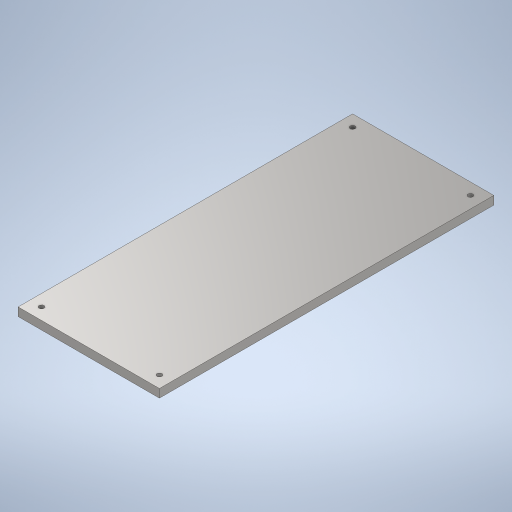
# Autodesk Inventor part: Tutup_system
Saved by Autodesk Inventor 2023.1 (Build 271208000, 208)
## iProperties
Created: 2024-03-27
Part Number: Tutup_system
Material: Generic
Document SubType Name: Modeling
Designer: bahariridwan
Density: 1 g/cm^3
Appearance: Stainless - Brushed
Author: bahariridwan
Autodesk Inventor part; units mm, degrees
ref_plane "YZ Plane" through (0, 0, 0) normal (1, 0, 0) x (0, 1, 0)
ref_plane "XZ Plane" through (0, 0, 0) normal (0, 1, 0) x (-1, 0, 0)
ref_plane "XY Plane" through (0, 0, 0) normal (0, 0, 1) x (1, 0, 0)
sketch "Sketch1" plane through (0, 0, 0) normal (0, 1, 0) x (-1, 0, 0)
  line L0 (0, 0) -> (84.487, 0)
  line L1 (84.487, 0) -> (84.487, -200)
  line L2 (84.487, -200) -> (0, -200)
  line L3 (0, -200) -> (0, 0)
  constraints: 8 end point, 2 parallel, 1 horizontal, 1 perpendicular
extrude "Extrusion1" add sketch "Sketch1" along normal blind 5
sketch "Sketch2" plane through (0, 5, 0) normal (0, 1, 0) x (1, 0, 0)
  circle A0 centre (-7, 7) radius 1.5
  circle A1 centre (-77.487, 7) radius 1.5
  circle A2 centre (-77.487, 193) radius 1.5
  circle A3 centre (-7, 193) radius 1.5
  line L0 (-84.487, 200) -> (-84.487, 0) projected
  line L1 (-84.487, 0) -> (0, 0) projected
  line L2 (0, 0) -> (0, 200) projected
  line L3 (0, 200) -> (-84.487, 200) projected
  dimension "d4" = 3
  dimension "d5" = 3
  dimension "d6" = 3
  dimension "d7" = 3
  dimension "d8" = 7
  dimension "d9" = 7
  dimension "d10" = 7
  dimension "d11" = 7
  dimension "d12" = 7
  dimension "d13" = 7
  dimension "d14" = 7
  dimension "d15" = 7
  constraints: 4 centre point
  measures "d4" diameter of A0
  measures "d5" diameter of A1
  measures "d6" diameter of A2
  measures "d7" diameter of A3
  measures "d8" distance from line of L0 A1.centre
  measures "d9" distance from line of L1 A1.centre
  measures "d10" distance from line of L2 A0.centre
  measures "d11" distance from line of L1 A0.centre
  measures "d12" distance from line of L0 A2.centre
  measures "d13" distance from line of L3 A2.centre
  measures "d14" distance from line of L2 A3.centre
  measures "d15" distance from line of L3 A3.centre
extrude "Extrusion2" cut sketch "Sketch2" against normal blind 5 contours A0 | A1 | A2 | A3
equation "\"d9\" = d8"
equation "\"d10\" = d8"
equation "\"d11\" = d8"
equation "\"d12\" = d8"
equation "\"d13\" = d8"
equation "\"d14\" = d8"
equation "\"d15\" = d8"
body "Solid1"
